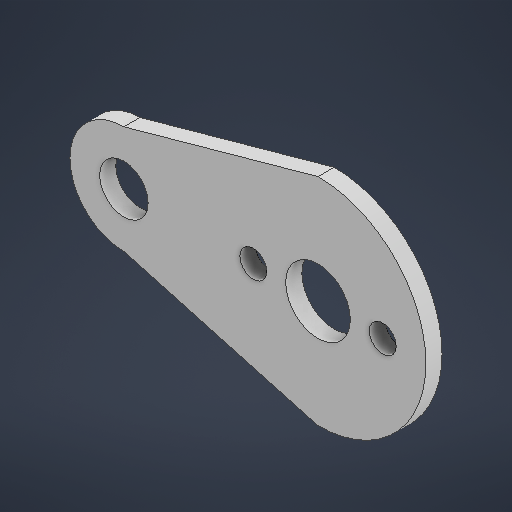
# Autodesk Inventor part: captorTest
Saved by Autodesk Inventor 2026.1 (Build 301233000, 233)
## iProperties
Created: 2026-01-27
Part Number: captorTest
Material: Generic
Document SubType Name: Modeling
Designer: fheli
Density: 1 g/cm^3
Appearance: Default
Author: fheli
Autodesk Inventor part; units mm, degrees
ref_plane "YZ Plane" through (0, 0, 0) normal (1, 0, 0) x (0, 1, 0)
ref_plane "XZ Plane" through (0, 0, 0) normal (0, 1, 0) x (-1, 0, 0)
ref_plane "XY Plane" through (0, 0, 0) normal (0, 0, 1) x (1, 0, 0)
sketch "Sketch1" plane through (0, 0, 0) normal (0, 0, 1) x (1, 0, 0)
  circle A0 centre (0, 0) radius 6
  circle A1 centre (0, 0) radius 20
  line L0 (0, 0) -> (12, 0)
  line L1 (0, 0) -> (-12, 0)
  circle A2 centre (-12, 0) radius 2.5
  circle A3 centre (12, 0) radius 2.5
  line L2 (0, 0) -> (-36, 0)
  circle A4 centre (-36, 0) radius 4.5
  circle A5 centre (-36, 0) radius 10
  line L3 (-36, 10) -> (0, 20)
  line L4 (-36, -10) -> (0, -20)
  dimension "d0" = 12
  dimension "d1" = 40
  dimension "d2" = 12
  dimension "d3" = 12
  dimension "d4" = 5
  dimension "d5" = 5
  dimension "d6" = 36
  dimension "d7" = 9
  dimension "d8" = 20
  constraints: 10 end point, 6 centre point, 6 coincident, 4 point on circle, 3 horizontal
  measures "d0" diameter of A0
  measures "d1" diameter of A1
  measures "d2" distance of L0.start L0.end
  measures "d3" distance of L0.start L1.end
  measures "d4" diameter of A2
  measures "d5" diameter of A3
  measures "d6" distance of L0.start L2.end
  measures "d7" diameter of A4
  measures "d8" diameter of A5
extrude "Extrusion1" add sketch "Sketch1" along normal blind 3 contours A1 L3 L4 | A1 L4 A5 L2 | L2 A5 L3 A1 | A5
body "Solid1"
